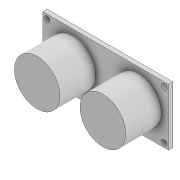
# Autodesk Inventor part: US-015
Saved by Autodesk Inventor 2022 (Build 260153000, 153)
## iProperties
Created: 2024-06-19
Part Number: US-015
Material: Generic
Document SubType Name: Modeling
Designer: david
Density: 1 g/cm^3
Appearance: Default
Author: david
Autodesk Inventor part; units mm, degrees
ref_plane "YZ Plane" through (0, 0, 0) normal (1, 0, 0) x (0, 1, 0)
ref_plane "XZ Plane" through (0, 0, 0) normal (0, 1, 0) x (-1, 0, 0)
ref_plane "XY Plane" through (0, 0, 0) normal (0, 0, 1) x (1, 0, 0)
sketch "Sketch1" plane through (0, 0, 0) normal (0, 0, 1) x (1, 0, 0)
  line L0 (-22, 20) -> (22, 20)
  line L1 (22, 20) -> (22, 0)
  line L2 (22, 0) -> (-22, 0)
  line L3 (-22, 0) -> (-22, 20)
  line L4 (-22, 20) -> (22, 0) construction
  line L5 (22, 20) -> (-22, 0) construction
  point P0 (0, 0)
  point P1 (0, 10)
  point P2 (0, 10)
  dimension "d0" = 44
  dimension "d1" = 20
  constraints: 12 end point, 4 midpoint, 2 parallel, 1 horizontal, 1 perpendicular, 1 vertical alignment
  measures "d0" distance of L1.end L2.end
  measures "d1" distance of L0.end L1.end
extrude "Extrusion1" add sketch "Sketch1" along normal blind 1.5
sketch "Sketch2" plane through (0, 0, 1.5) normal (0, 0, 1) x (1, 0, 0)
  circle A0 centre (-11.5, 10) radius 8
  line L0 (0, -4) -> (0, 24) projected
  circle A1 centre (11.5, 10) radius 8
  line L1 (-22, 20) -> (-22, 0) projected
  point P0 (0, 0)
  point P1 (-22, 10)
  point P2 (-19.5, 10)
  dimension "d4" = 16
  dimension "d5" = 2.5
  constraints: 3 horizontal alignment, 1 centre point, 1 midpoint, 1 symmetric about line, 3 other
  measures "d4" diameter of A1
  measures "d5" distance of point (-22, 10) point (-19.5, 10)
extrude "Extrusion2" add sketch "Sketch2" along normal blind 12.5
sketch "Sketch3" plane through (0, 0, 0) normal (0, 0, -1) x (-1, 0, 0)
  line L0 (21.5, 19.5) -> (-21.5, 19.5)
  line L1 (-21.5, 19.5) -> (-21.5, 0.5)
  line L2 (-21.5, 0.5) -> (21.5, 0.5)
  line L3 (21.5, 0.5) -> (21.5, 19.5)
  line L4 (21.5, 19.5) -> (-21.5, 0.5) construction
  line L5 (-21.5, 19.5) -> (21.5, 0.5) construction
  line L6 (-22, 0) -> (-22, 20) projected
  line L7 (-22, 20) -> (22, 20) projected
  line L8 (22, 20) -> (22, 0) projected
  line L9 (22, 0) -> (-22, 0) projected
  circle A0 centre (-20.5, 18.5) radius 1
  circle A1 centre (-20.5, 1.5) radius 1
  circle A2 centre (20.5, 18.5) radius 1
  circle A3 centre (20.5, 1.5) radius 1
  point P0 (0, 0)
  point P1 (0, 10)
  dimension "d8" = 0.5
  dimension "d9" = 0.5
  dimension "d10" = 0.5
  dimension "d11" = 0.5
  dimension "d12" = 2
  dimension "d13" = 2
  dimension "d14" = 2
  dimension "d15" = 2
  constraints: 12 end point, 8 tangent, 4 centre point, 4 coincident, 2 midpoint, 2 parallel, 1 horizontal, 1 perpendicular
  measures "d8" distance between parallel lines of L6 L1
  measures "d9" distance between parallel lines of L0 L7
  measures "d10" distance between parallel lines of L3 L8
  measures "d11" distance between parallel lines of L9 L2
  measures "d12" diameter of A0
  measures "d13" diameter of A1
  measures "d14" diameter of A2
  measures "d15" diameter of A3
hole "Hole1" at (-20.5, 1.5, 0) at (-20.5, 18.5, 0) at (20.5, 1.5, 0) at (20.5, 18.5, 0) direction (0, 0, 1) diameter 2 depth 6
equation "\"d10\" = d8"
equation "\"d11\" = d9"
equation "\"d13\" = d14"
equation "\"d14\" = d12"
equation "\"d15\" = d12"
equation "\"d16\" = d12"
body "Solid1"
